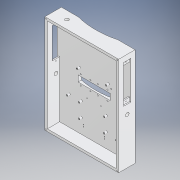
# Autodesk Inventor part: BP001b
Saved by Autodesk Inventor 2017 SP1 (Build 210196100, 196)
## iProperties
Created: 2017-12-18
Part Number: BP001b
Material: ABS Plastic
Document SubType Name: Modeling
Designer: Zach
Density: 1.06 g/cm^3
Appearance: CR White
Author: Zach
Autodesk Inventor part; units mm, degrees
ref_plane "YZ Plane" through (0, 0, 0) normal (1, 0, 0) x (0, 1, 0)
ref_plane "XZ Plane" through (0, 0, 0) normal (0, 1, 0) x (-1, 0, 0)
ref_plane "XY Plane" through (0, 0, 0) normal (0, 0, 1) x (1, 0, 0)
sketch "Sketch1" plane through (0, 0, 0) normal (0, 0, 1) x (1, 0, 0)
  line L0 (0, 0) -> (130, 0)
  line L1 (130, 0) -> (130, 25)
  line L2 (130, 25) -> (0, 25)
  line L3 (0, 25) -> (0, 0)
  line L4 (10.3559, 32.5) -> (50.3559, 32.5) construction
  line L5 (50.3559, 32.5) -> (50.3559, -7.5) construction
  line L6 (50.3559, -7.5) -> (10.3559, -7.5) construction
  line L7 (10.3559, -7.5) -> (10.3559, 32.5) construction
  line L8 (79.6441, 32.5) -> (119.6441, 32.5) construction
  line L9 (119.6441, 32.5) -> (119.6441, -7.5) construction
  line L10 (119.6441, -7.5) -> (79.6441, -7.5) construction
  line L11 (79.6441, -7.5) -> (79.6441, 32.5) construction
  line L12 (50.3559, 12.5) -> (79.6441, 12.5) construction
  circle A0 centre (10.3559, 32.5) radius 2.5
  circle A1 centre (50.3559, 32.5) radius 2.5
  circle A2 centre (50.3559, -7.5) radius 2.5
  circle A3 centre (10.3559, -7.5) radius 2.5
  circle A4 centre (79.6441, -7.5) radius 2.5
  circle A5 centre (119.6441, -7.5) radius 2.5
  circle A6 centre (119.6441, 32.5) radius 2.5
  circle A7 centre (79.6441, 32.5) radius 2.5
  line L13 (-85, -187.5) -> (215, -187.5)
  line L14 (215, -187.5) -> (215, 212.5)
  line L15 (215, 212.5) -> (-85, 212.5)
  line L16 (-85, 212.5) -> (-85, -187.5)
  point P0 (130, 12.5)
  point P1 (65, 12.5)
  point P2 (65, 25)
  point P3 (215, 12.5)
  point P4 (65, 212.5)
  dimension "d0" = 130
  dimension "d1" = 25
  dimension "d2" = 40
  dimension "d3" = 40
  dimension "d4" = 40
  dimension "d5" = 40
  dimension "d6" = 29.2883
  dimension "d7" = 5
  dimension "d8" = 5
  dimension "d9" = 5
  dimension "d10" = 5
  dimension "d11" = 5
  dimension "d12" = 5
  dimension "d13" = 5
  dimension "d14" = 5
  dimension "d15" = 300
  dimension "d16" = 400
  constraints: 34 end point, 8 centre point, 8 coincident, 8 parallel, 7 midpoint, 4 horizontal, 4 perpendicular, 2 horizontal alignment, 2 vertical alignment, 1 point on line
  measures "d0" distance of L2.end L1.end
  measures "d1" distance of L1.end L0.end
  measures "d2" distance of L5.end L6.end
  measures "d3" distance of L4.end L5.end
  measures "d4" distance of L9.end L10.end
  measures "d5" distance of L8.end L9.end
  measures "d6" distance between parallel lines of L11 L5
  measures "d7" diameter of A0
  measures "d8" diameter of A1
  measures "d9" diameter of A2
  measures "d10" diameter of A3
  measures "d11" diameter of A4
  measures "d12" diameter of A5
  measures "d13" diameter of A6
  measures "d14" diameter of A7
  measures "d15" distance of L15.end L14.end
  measures "d16" distance of L14.end L13.end
extrude "Extrusion1" add sketch "Sketch1" along normal blind 17
sketch "Sketch2" plane through (0, 0, 17) normal (0, 0, 1) x (1, 0, 0)
  line L0 (-85, 212.5) -> (-85, -187.5) projected
  line L1 (215, 212.5) -> (-85, 212.5) projected
  line L2 (215, -187.5) -> (215, 212.5) projected
  line L3 (-85, -187.5) -> (215, -187.5) projected
  line L4 (-75, -177.5) -> (-75, 202.5)
  line L5 (-75, 202.5) -> (205, 202.5)
  line L6 (205, 202.5) -> (205, -177.5)
  line L7 (205, -177.5) -> (-75, -177.5)
  point P0 (0, 0)
  dimension "d19" = 10
  constraints: 8 end point, 3 other
  measures "d19" distance between parallel lines of L0 L4
extrude "Extrusion2" add sketch "Sketch2" along normal blind 50
sketch "Sketch3" plane through (-85, 212.5, 0) normal (0, 1, 0) x (1, 0, 0)
  line L0 (0, 0) -> (300, 0) construction
  line L1 (70, 0) -> (230, 0)
  arc A0 (70, 0) -> (230, 0) centre (150, 304.672) ccw
  point P0 (85, 0)
  point P1 (150, 0)
  dimension "d23" = 160
  dimension "d24" = 315
  constraints: 2 end point, 2 midpoint, 2 point on circle, 2 point on line, 1 centre point
  measures "d23" distance of L1.start L1.end
  measures "d24" radius of A0
extrude "Extrusion3" cut sketch "Sketch3" against normal through all
sketch "Sketch5" plane through (0, 0, 17) normal (0, 0, 1) x (1, 0, 0)
  line L0 (6.5, 172.25) -> (123.5, 172.25) construction
  line L1 (123.5, 172.25) -> (123.5, 55.25) construction
  line L2 (123.5, 55.25) -> (6.5, 55.25) construction
  line L3 (6.5, 55.25) -> (6.5, 172.25) construction
  line L4 (0, 25) -> (130, 25) construction
  line L5 (65, 25) -> (65, 202.5) construction
  line L6 (-75, 202.5) -> (205, 202.5) construction
  circle A0 centre (123.5, 172.25) radius 1.5
  circle A1 centre (123.5, 55.25) radius 1.5
  circle A2 centre (6.5, 55.25) radius 1.5
  circle A3 centre (6.5, 172.25) radius 1.5
  line L7 (37, -38.75) -> (93, -38.75) construction
  circle A4 centre (93, -38.75) radius 1.5
  circle A5 centre (37, -38.75) radius 1.5
  line L8 (130, 0) -> (0, 0) construction
  line L9 (65, 0) -> (65, -177.5) construction
  line L10 (-75, -177.5) -> (205, -177.5) projected
  line L11 (22.5, -146.75) -> (107.5, -146.75) construction
  line L12 (107.5, -146.75) -> (107.5, -138.75) construction
  line L13 (107.5, -138.75) -> (22.5, -138.75) construction
  line L14 (22.5, -138.75) -> (22.5, -146.75) construction
  circle A6 centre (107.5, -138.75) radius 1.5
  circle A7 centre (107.5, -146.75) radius 1.5
  circle A8 centre (22.5, -138.75) radius 1.5
  circle A9 centre (22.5, -146.75) radius 1.5
  line L15 (93, -38.75) -> (93, -138.75) construction
  line L16 (-35, -59.75) -> (14, -59.75) construction
  line L17 (14, -59.75) -> (14, -117.75) construction
  line L18 (14, -117.75) -> (-35, -117.75) construction
  line L19 (-35, -117.75) -> (-35, -59.75) construction
  circle A10 centre (-35, -59.75) radius 1.5
  circle A11 centre (14, -59.75) radius 1.5
  circle A12 centre (14, -117.75) radius 1.5
  line L20 (-75, -177.5) -> (-75, 202.5) projected
  line L21 (116, -59.75) -> (165, -59.75) construction
  line L22 (165, -59.75) -> (165, -117.75) construction
  line L23 (165, -117.75) -> (116, -117.75) construction
  line L24 (116, -117.75) -> (116, -59.75) construction
  line L25 (205, 202.5) -> (205, -177.5) projected
  circle A13 centre (165, -117.75) radius 1.5
  circle A14 centre (116, -117.75) radius 1.5
  circle A15 centre (116, -59.75) radius 1.5
  point P0 (65, 55.25)
  point P1 (65, 113.75)
  point P2 (123.5, 113.75)
  point P3 (65, -38.75)
  point P4 (65, -138.75)
  point P5 (93, -88.75)
  point P6 (14, -88.75)
  point P7 (65, -88.75)
  point P8 (116, -88.75)
  dimension "d27" = 117
  dimension "d28" = 117
  dimension "d29" = 3
  dimension "d30" = 3
  dimension "d31" = 3
  dimension "d32" = 3
  dimension "d33" = 56
  dimension "d34" = 3
  dimension "d35" = 3
  dimension "d36" = 85
  dimension "d37" = 8
  dimension "d38" = 3
  dimension "d39" = 3
  dimension "d40" = 3
  dimension "d41" = 3
  dimension "d42" = 100
  dimension "d43" = 49
  dimension "d44" = 58
  dimension "d45" = 3
  dimension "d46" = 3
  dimension "d48" = 3
  dimension "d49" = 40
  dimension "d50" = 49
  dimension "d51" = 58
  dimension "d52" = 40
  dimension "d53" = 3
  dimension "d54" = 3
  dimension "d55" = 3
  constraints: 40 end point, 16 centre point, 16 coincident, 13 midpoint, 8 parallel, 5 horizontal, 4 horizontal alignment, 4 perpendicular, 3 point on line, 1 vertical, 1 vertical alignment
  measures "d27" distance of L1.end L2.end
  measures "d28" distance of L0.end L1.end
  measures "d29" diameter of A0
  measures "d30" diameter of A1
  measures "d31" diameter of A2
  measures "d32" diameter of A3
  measures "d33" distance of L7.start L7.end
  measures "d34" diameter of A4
  measures "d35" diameter of A5
  measures "d36" distance of L13.end L12.end
  measures "d37" distance of L12.end L11.end
  measures "d38" diameter of A6
  measures "d39" diameter of A7
  measures "d40" diameter of A8
  measures "d41" diameter of A9
  measures "d42" distance of L15.start L15.end
  measures "d43" distance of L17.end L18.end
  measures "d44" distance of L16.end L17.end
  measures "d45" diameter of A10
  measures "d46" diameter of A11
  measures "d48" diameter of A12
  measures "d49" distance between parallel lines of L20 L19
  measures "d50" distance of L22.end L23.end
  measures "d51" distance of L21.end L22.end
  measures "d52" distance between parallel lines of L25 L22
  measures "d53" diameter of A13
  measures "d54" diameter of A14
  measures "d55" diameter of A15
extrude "Extrusion4" cut sketch "Sketch5" against normal through all
sketch "Sketch6" plane through (0, 0, 17) normal (0, 0, 1) x (1, 0, 0)
  circle A0 centre (6.5, 172.25) radius 1.5 projected
  circle A1 centre (116, -117.75) radius 1.5 projected
  circle A2 centre (14, -117.75) radius 1.5 projected
  circle A3 centre (-35, -59.75) radius 1.5 projected
  circle A4 centre (22.5, -138.75) radius 1.5 projected
  circle A5 centre (107.5, -138.75) radius 1.5 projected
  circle A6 centre (93, -38.75) radius 1.5 projected
  circle A7 centre (6.5, 55.25) radius 1.5 projected
  circle A8 centre (123.5, 172.25) radius 1.5 projected
  circle A9 centre (123.5, 55.25) radius 1.5 projected
  circle A10 centre (6.5, 172.25) radius 1.5 projected
  circle A11 centre (37, -38.75) radius 1.5 projected
  circle A12 centre (107.5, -146.75) radius 1.5 projected
  circle A13 centre (22.5, -146.75) radius 1.5 projected
  circle A14 centre (14, -59.75) radius 1.5 projected
  circle A15 centre (165, -117.75) radius 1.5 projected
  circle A16 centre (116, -59.75) radius 1.5 projected
  line L0 (205, 202.5) -> (-75, 202.5) projected
  line L1 (-75, 202.5) -> (-75, -177.5) projected
  line L2 (-75, -177.5) -> (205, -177.5) projected
  line L3 (205, -177.5) -> (205, 202.5) projected
  line L4 (0, 0) -> (0, 25) projected
  line L5 (0, 25) -> (130, 25) projected
  line L6 (130, 25) -> (130, 0) projected
  line L7 (130, 0) -> (0, 0) projected
  circle A17 centre (79.6441, 32.5) radius 2.5 projected
  circle A18 centre (119.6441, 32.5) radius 2.5 projected
  circle A19 centre (119.6441, -7.5) radius 2.5 projected
  circle A20 centre (79.6441, -7.5) radius 2.5 projected
  circle A21 centre (10.3559, -7.5) radius 2.5 projected
  circle A22 centre (50.3559, -7.5) radius 2.5 projected
  circle A23 centre (50.3559, 32.5) radius 2.5 projected
  circle A24 centre (10.3559, 32.5) radius 2.5 projected
  circle A25 centre (6.5, 172.25) radius 3.5
  circle A26 centre (123.5, 172.25) radius 1.5 projected
  circle A27 centre (123.5, 172.25) radius 3.5
  circle A28 centre (123.5, 55.25) radius 3.5
  circle A29 centre (6.5, 55.25) radius 1.5 projected
  circle A30 centre (6.5, 55.25) radius 3.5
  circle A31 centre (-35, -59.75) radius 3.5
  circle A32 centre (14, -59.75) radius 1.5 projected
  circle A33 centre (14, -59.75) radius 3.5
  circle A34 centre (14, -117.75) radius 1.5 projected
  circle A35 centre (14, -117.75) radius 3.5
  circle A36 centre (116, -59.75) radius 1.5 projected
  circle A37 centre (116, -59.75) radius 3.5
  circle A38 centre (116, -117.75) radius 1.5 projected
  circle A39 centre (116, -117.75) radius 3.5
  circle A40 centre (165, -117.75) radius 3.5
  dimension "d58" = 7
  dimension "d59" = 7
  dimension "d60" = 7
  dimension "d61" = 7
  dimension "d62" = 7
  dimension "d63" = 7
  dimension "d64" = 7
  dimension "d65" = 7
  dimension "d66" = 7
  dimension "d67" = 7
  constraints: 10 centre point, 10 coincident
  measures "d58" diameter of A25
  measures "d59" diameter of A27
  measures "d60" diameter of A28
  measures "d61" diameter of A30
  measures "d62" diameter of A31
  measures "d63" diameter of A33
  measures "d64" diameter of A35
  measures "d65" diameter of A37
  measures "d66" diameter of A39
  measures "d67" diameter of A40
extrude "Extrusion5" add sketch "Sketch6" along normal blind 10 contours A25 | A27 | A28 | A30 | A31 | A33 | A35 | A37 | A39 | A40
sketch "Sketch7" plane through (-75, -177.5, 17) normal (1, 0, 0) x (0, 0, -1)
  line L0 (-10, 353.25) -> (-10, 346.25) projected
  line L1 (0, 346.25) -> (0, 353.25) projected
  line L2 (-10, 236.25) -> (-10, 229.25) projected
  line L3 (0, 229.25) -> (0, 236.25) projected
  line L4 (0, 353.25) -> (-30, 353.25)
  line L5 (-30, 353.25) -> (-30, 229.25)
  line L6 (-30, 229.25) -> (0, 229.25)
  line L7 (0, 229.25) -> (0, 353.25)
  point P0 (17, 177.5)
  dimension "d70" = 30
  constraints: 8 end point, 2 parallel, 1 horizontal, 1 perpendicular
  measures "d70" distance between parallel lines of L7 L5
extrude "Extrusion6" cut sketch "Sketch7" against normal through all
sketch "Sketch8" plane through (-85, -187.5, 0) normal (-1, 0, 0) x (0, 0, 1)
  line L0 (47, 363.25) -> (47, 239.25) projected
  line L1 (17, 239.25) -> (17, 363.25) projected
  line L2 (47, 363.25) -> (17, 363.25)
  line L3 (17, 363.25) -> (17, 378.25)
  line L4 (17, 378.25) -> (47, 378.25)
  line L5 (47, 378.25) -> (47, 363.25)
  line L6 (47, 239.25) -> (17, 239.25)
  line L7 (17, 239.25) -> (17, 224.25)
  line L8 (17, 224.25) -> (47, 224.25)
  line L9 (47, 224.25) -> (47, 239.25)
  point P0 (0, 187.5)
  dimension "d73" = 15
  dimension "d74" = 15
  constraints: 16 end point, 4 parallel, 2 horizontal, 2 perpendicular
  measures "d73" distance of L1.end L3.end
  measures "d74" distance of L1.start L7.end
extrude "Extrusion7" cut sketch "Sketch8" against normal blind 5 contours L2 L3 L4 L5 | L9 L8 L7 L6
sketch "Sketch9" plane through (-80, -187.5, 0) normal (-1, 0, 0) x (0, 0, 1)
  circle A0 centre (32, 231.75) radius 1.5
  line L0 (17, 239.25) -> (47, 239.25) projected
  line L1 (17, 224.25) -> (17, 239.25) projected
  line L2 (47, 224.25) -> (17, 224.25) projected
  line L3 (47, 239.25) -> (47, 224.25) projected
  line L4 (17, 378.25) -> (47, 378.25) projected
  line L5 (47, 378.25) -> (47, 363.25) projected
  line L6 (17, 378.25) -> (47, 378.25) projected
  line L7 (17, 363.25) -> (17, 378.25) projected
  line L8 (47, 363.25) -> (17, 363.25) projected
  circle A1 centre (32, 370.75) radius 1.5
  point P0 (0, 187.5)
  point P1 (17, 231.75)
  point P2 (32, 239.25)
  point P3 (17, 370.75)
  point P4 (32, 363.25)
  dimension "d77" = 3
  dimension "d78" = 3
  constraints: 4 midpoint, 2 centre point, 2 horizontal alignment, 2 vertical alignment
  measures "d77" diameter of A0
  measures "d78" diameter of A1
extrude "Extrusion8" cut sketch "Sketch9" against normal through all contours A0 | A1
sketch "Sketch10" plane through (215, -187.5, 0) normal (1, 0, 0) x (0, 0, -1)
  line L0 (-47, 363.25) -> (-17, 363.25)
  line L1 (-47, 363.25) -> (-17, 363.25)
  line L2 (-17, 363.25) -> (-17, 378.25)
  line L3 (-17, 378.25) -> (-47, 378.25)
  line L4 (-47, 378.25) -> (-47, 363.25)
  line L5 (-47, 239.25) -> (-17, 239.25)
  line L6 (-47, 239.25) -> (-17, 239.25)
  line L7 (-17, 239.25) -> (-17, 224.25)
  line L8 (-17, 224.25) -> (-47, 224.25)
  line L9 (-47, 224.25) -> (-47, 239.25)
  line L10 (-47, 239.25) -> (-47, 363.25) projected
  line L11 (-17, 239.25) -> (-47, 239.25) projected
  line L12 (-47, 363.25) -> (-17, 363.25) projected
  point P0 (0, 187.5)
  dimension "d81" = 15
  dimension "d83" = 15
  constraints: 20 end point, 4 parallel, 2 horizontal, 2 perpendicular
  measures "d81" distance of L0.end L2.end
  measures "d83" distance of L5.end L7.end
extrude "Extrusion9" cut sketch "Sketch10" against normal blind 5
sketch "Sketch11" plane through (-75, -177.5, 67) normal (1, 0, 0) x (0, 0, -1)
  circle A0 centre (35, 177.5) radius 7.5
  line L0 (50, 229.25) -> (20, 229.25) projected
  point P0 (67, 177.5)
  point P1 (35, 229.25)
  dimension "d86" = 15
  constraints: 1 centre point, 1 horizontal alignment, 1 midpoint, 1 vertical alignment
  measures "d86" diameter of A0
extrude "Extrusion10" cut sketch "Sketch11" along normal through all both and the other way through all
sketch "Sketch12" plane through (0, 0, 17) normal (0, 0, 1) x (1, 0, 0)
  line L0 (-5, 183.75) -> (135, 183.75) construction
  line L1 (135, 183.75) -> (135, 43.75) construction
  line L2 (135, 43.75) -> (-5, 43.75) construction
  line L3 (-5, 43.75) -> (-5, 183.75) construction
  circle A0 centre (7, 185.13) radius 1.5 construction
  circle A1 centre (7, 42.37) radius 1.5 construction
  circle A2 centre (123, 185.13) radius 1.5 construction
  circle A3 centre (-5, 43.75) radius 2.5
  circle A4 centre (135, 43.75) radius 2.5
  circle A5 centre (135, 183.75) radius 2.5
  circle A6 centre (-5, 183.75) radius 2.5
  circle A7 centre (6.5, 172.25) radius 1.5 projected
  circle A8 centre (6.5, 55.25) radius 1.5 projected
  circle A9 centre (123.5, 55.25) radius 1.5 projected
  line L4 (6.5, 172.25) -> (6.5, 55.25) construction
  line L5 (6.5, 55.25) -> (123.5, 55.25) construction
  point P0 (0, 0)
  point P1 (135, 113.75)
  point P2 (6.5, 113.75)
  point P3 (-5, 113.75)
  point P4 (65, 55.25)
  point P5 (65, 43.75)
  dimension "d89" = 140
  dimension "d90" = 140
  dimension "d91" = 5
  dimension "d92" = 5
  dimension "d93" = 5
  dimension "d94" = 5
  constraints: 12 end point, 7 centre point, 5 midpoint, 4 coincident, 2 parallel, 2 perpendicular, 1 horizontal, 1 horizontal alignment, 1 vertical, 1 vertical alignment
  measures "d89" distance of L1.end L2.end
  measures "d90" distance of L0.end L1.end
  measures "d91" diameter of A3
  measures "d92" diameter of A4
  measures "d93" diameter of A5
  measures "d94" diameter of A6
extrude "Extrusion11" cut sketch "Sketch12" against normal through all contours A3 | A4 | A5 | A6
sketch "Sketch13" plane through (205, -177.5, 17) normal (-1, 0, 0) x (0, 0, 1)
  line L0 (30, 353.25) -> (0, 353.25) projected
  circle A0 centre (15, 177.5) radius 7.5 projected
  circle A1 centre (15, 221.75) radius 1.5 projected
  circle A2 centre (15, 360.75) radius 1.5 projected
  line L1 (0, 0) -> (0, 380) projected
  line L2 (0, 0) -> (50, 0) projected
  line L3 (0, 229.25) -> (30, 229.25) projected
  line L4 (0, 353.25) -> (30, 353.25) projected
  line L5 (30, 353.25) -> (30, 229.25)
  line L6 (0, 229.25) -> (0, 214.25) projected
  line L7 (0, 229.25) -> (0, 353.25)
  point P0 (-17, 177.5)
  constraints: 4 end point, 3 centre point, 1 collinear, 1 perpendicular
extrude "Extrusion12" cut sketch "Sketch13" against normal through all contours L5 L3 L1 L0
sketch "Sketch14" plane through (-85, 212.5, 67) normal (0, 1, 0) x (1, 0, 0)
  line L0 (290, 50) -> (10, 50) projected
  circle A0 centre (55, 35) radius 7.5
  line L1 (150, 50) -> (150, -11.8542)
  point P0 (85, 67)
  dimension "d99" = 15
  dimension "d100" = 15
  dimension "d103" = 95
  constraints: 2 end point, 1 centre point, 1 midpoint, 1 vertical
  measures "d99" diameter of A0
  measures "d100" distance from line of L0 A0.centre
  measures "d103" distance from line of L1 A0.centre
extrude "Extrusion13" cut sketch "Sketch14" against normal blind 25
sketch "Sketch15" plane through (0, 0, 67) normal (0, 0, 1) x (1, 0, 0)
  line L0 (-75, 202.5) -> (205, 202.5) construction
  line L1 (205, 202.5) -> (205, -177.5) construction
  line L2 (205, -177.5) -> (-75, -177.5) construction
  line L3 (-75, -177.5) -> (-75, 202.5) construction
  line L4 (-85, 212.5) -> (-85, -187.5) construction
  line L5 (-85, -187.5) -> (215, -187.5) construction
  line L6 (215, -187.5) -> (215, 212.5) construction
  line L7 (215, 212.5) -> (-85, 212.5) construction
  line L8 (-80, 207.5) -> (-80, -182.5) construction
  line L9 (-80, -182.5) -> (210, -182.5) construction
  line L10 (210, -182.5) -> (210, 207.5) construction
  line L11 (210, 207.5) -> (-80, 207.5) construction
  circle A0 centre (-80, 207.5) radius 2.5
  circle A1 centre (210, 207.5) radius 2.5
  circle A2 centre (210, -182.5) radius 2.5
  circle A3 centre (-80, -182.5) radius 2.5
  point P0 (0, 0)
  dimension "d105" = 5
  dimension "d106" = 5
  dimension "d107" = 5
  dimension "d108" = 5
  dimension "d109" = 5
  constraints: 8 end point, 4 centre point, 4 coincident, 3 other
  measures "d105" distance between parallel lines of L7 L11
  measures "d106" diameter of A0
  measures "d107" diameter of A1
  measures "d108" diameter of A2
  measures "d109" diameter of A3
extrude "Extrusion14" cut sketch "Sketch15" against normal blind 25
body "Solid1"
